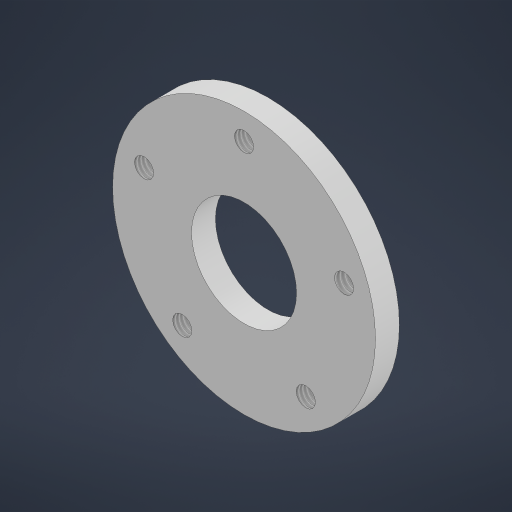
# Autodesk Inventor part: panel_flange
Saved by Autodesk Inventor 2023.2 (Build 272271030, 271C)
## iProperties
Created: 2023-11-12
Part Number: panel_flange
Material: Generic
Document SubType Name: Modeling
Designer: ralph
Density: 1 g/cm^3
Appearance: Default
Author: ralph
Autodesk Inventor part; units mm, degrees
ref_plane "YZ Plane" through (0, 0, 0) normal (1, 0, 0) x (0, 1, 0)
ref_plane "XZ Plane" through (0, 0, 0) normal (0, 1, 0) x (-1, 0, 0)
ref_plane "XY Plane" through (0, 0, 0) normal (0, 0, 1) x (1, 0, 0)
sketch "Sketch1" plane through (0, 0, 0) normal (0, 0, 1) x (1, 0, 0)
  circle A0 centre (0, 0) radius 13.97
  circle A1 centre (0, 0) radius 34.925
  circle A2 centre (0, 0) radius 27.94
  point P0 (0, 27.94)
  point P1 (-26.5725, 8.6339)
  point P2 (-16.4227, -22.6039)
  point P3 (16.4227, -22.6039)
  point P4 (26.5725, 8.6339)
  dimension "d2" = 55.88
  dimension "d0" = 27.94
  dimension "d1" = 69.85
  dimension "d5" = 360
  constraints: 5 coincident, 2 centre point, 1 vertical alignment, 11 other
  measures "d0" diameter of A0
  measures "d1" diameter of A1
extrude "Extrusion1" add sketch "Sketch1" along normal blind 6.35 contours A1 | A2
hole "Hole1" at (0, 27.94, 0) at (-26.5725, 8.6339, 0) at (-16.4227, -22.6039, 0) at (16.4227, -22.6039, 0) at (26.5725, 8.6339, 0) direction (0, 0, 1) diameter 5.1054 end through all
thread "Thread1" size "1/4-20 UNC" class "2B" standard "ANSI Unified Screw Threads" full length
thread "Thread2" size "12-24 UNC" class "2B" standard "ANSI Unified Screw Threads" full length
thread "Thread3" size "12-24 UNC" class "2B" standard "ANSI Unified Screw Threads" full length
thread "Thread4" size "12-24 UNC" class "2B" standard "ANSI Unified Screw Threads" full length
thread "Thread5" size "12-24 UNC" class "2B" standard "ANSI Unified Screw Threads" full length
body "Solid1"
